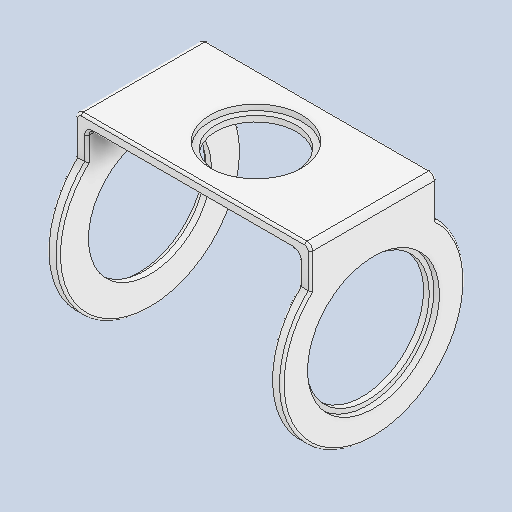
# Autodesk Inventor part: frame
Saved by Autodesk Inventor 2025.3 (Build 293356030, 356C)
## iProperties
Created: 2025-08-30
Part Number: frame
Material: PLA+ filament
Document SubType Name: Modeling
Designer: MSI
Density: 1.23 g/cm^3
Appearance: 일반
Mass: 632.221 g
Surface Area: 1234.42 cm^2
Volume: 514.001 cm^3
Author: MSI
Autodesk Inventor part; units mm, degrees
ref_plane "YZ Plane" through (0, 0, 0) normal (1, 0, 0) x (0, 1, 0)
ref_plane "XZ Plane" through (0, 0, 0) normal (0, 1, 0) x (-1, 0, 0)
ref_plane "XY Plane" through (0, 0, 0) normal (0, 0, 1) x (1, 0, 0)
sketch "스케치1" plane through (0, 0, 0) normal (1, 0, 0) x (0, 1, 0)
  circle A0 centre (0, 0) radius 80
  line L0 (0, 55) -> (93, 55)
  line L1 (93, 55) -> (93, -55)
  line L2 (93, -55) -> (0, -55)
  line L3 (0, -55) -> (0, 55)
  point P0 (58.0948, -55)
  point P1 (58.0948, 55)
  dimension "d0" = 160
  dimension "d1" = 93
  dimension "d36" = 110
  constraints: 8 end point, 3 coincident, 2 parallel, 1 centre point, 1 horizontal, 1 midpoint, 1 perpendicular
  measures "d0" diameter of A0
  measures "d1" distance of L1.end L2.end
  measures "d36" distance of L0.end L1.end
extrude "돌출1" add sketch "스케치1" along normal mid plane 205
sketch "스케치2" plane through (-102.5, 0, 55) normal (0, 0, 1) x (1, 0, 0)
  line L0 (10, 83) -> (195, 83)
  line L1 (195, 83) -> (195, -167)
  line L2 (195, -167) -> (10, -167)
  line L3 (10, -167) -> (10, 83)
  line L4 (205, 93) -> (0, 93) projected
  line L5 (0, 58.0948) -> (0, 93) projected
  point P0 (102.5, 0)
  point P1 (102.5, 0)
  point P2 (102.5, 83)
  dimension "d4" = 10
  dimension "d5" = 10
  dimension "d37" = 250
  constraints: 8 end point, 2 parallel, 1 coincident, 1 horizontal, 1 midpoint, 1 perpendicular, 1 vertical alignment
  measures "d4" distance between parallel lines of L0 L4
  measures "d5" distance between parallel lines of L5 L3
  measures "d37" distance of L2.end L0.start
extrude "돌출2" cut sketch "스케치2" along normal through all both and the other way through all
sketch "스케치4" plane through (-102.5, 93, 55) normal (0, 1, 0) x (1, 0, 0)
  point P0 (102.5, 55)
  point P1 (102.5, 55)
  constraints: 1 coincident
hole "구멍1" at (0, 93, 0) direction (0, -1, 0) diameter 70 end through all counterbore diameter 80 counterbore depth 5
sketch "스케치5" plane through (102.5, 0, 0) normal (1, 0, 0) x (0, 0, -1)
  arc A0 (-55, 58.0948) -> (55, 58.0948) centre (0, 0) ccw projected
  point P0 (-80, 0)
  constraints: 1 coincident
hole "구멍2" at (102.5, 0, 0) direction (-1, 0, 0) diameter 107.25 end through all counterbore diameter 115 counterbore depth 5
mirror "미러1" about plane through (0, 0, 0) normal (1, 0, 0) of "구멍2"
fillet "모깎기1" radius 5 2 edges at (-92.5, 83, 0) (92.5, 83, 0)
fillet "모깎기2" radius 5 2 edges at (-102.5, 93, 0) (102.5, 93, 0)
fillet "모깎기3" radius 2 24 edges at (-91.0355, 81.5355, 55) (0, 83, 55) (91.0355, 81.5355, 55) (92.5, 68.0474, 55) (92.5, -80, 0) (92.5, 68.0474, -55) (91.0355, 81.5355, -55) (0, 83, -55) (-91.0355, 81.5355, -55) (-92.5, 68.0474, -55) (-92.5, -80, 0) (-92.5, 68.0474, 55) (102.5, -80, 0) (102.5, 73.0474, -55) (101.0355, 91.5355, -55) (0, 93, -55) (-101.0355, 91.5355, -55) (-102.5, 73.0474, -55) (-102.5, -80, 0) (-102.5, 73.0474, 55) (-101.0355, 91.5355, 55) (0, 93, 55) (101.0355, 91.5355, 55) (102.5, 73.0474, 55)
equation "\"d5\" = d4"
